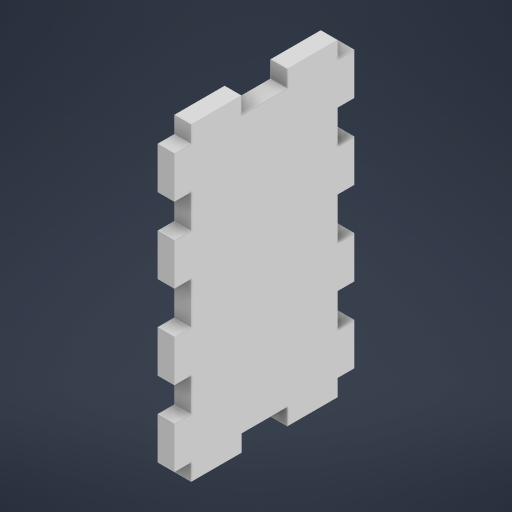
# Autodesk Inventor part: Langbektang houder
Saved by Autodesk Inventor 2023.2 (Build 272271000, 271)
## iProperties
Created: 2020-09-09
Part Number: Langbektang houder
Material: Generic
Document SubType Name: Modeling
Designer: nathan.bollaert
Density: 1 g/cm^3
Appearance: Default
Author: nathan.bollaert
Autodesk Inventor part; units mm, degrees
ref_plane "YZ Plane" through (0, 0, 0) normal (1, 0, 0) x (0, 1, 0)
ref_plane "XZ Plane" through (0, 0, 0) normal (0, 1, 0) x (-1, 0, 0)
ref_plane "XY Plane" through (0, 0, 0) normal (0, 0, 1) x (1, 0, 0)
sketch "Sketch1" plane through (0, 0, 0) normal (1, 0, 0) x (0, 1, 0)
  line L0 (0, 0) -> (74, 0)
  line L1 (74, 0) -> (74, -43)
  line L2 (74, -43) -> (0, -43)
  line L3 (0, -43) -> (0, 0)
  dimension "d228" = 74
  dimension "d229" = 43
  constraints: 8 end point, 2 parallel, 1 horizontal, 1 perpendicular
  measures "d228" distance of L1.end L2.end
  measures "d229" distance of L0.end L1.end
extrude "Extrusion1" add sketch "Sketch1" against normal blind 4
sketch "Sketch15" plane through (0, 0, 0) normal (1, 0, 0) x (0, 0, -1)
  line L0 (0, 74) -> (43, 74) projected
  line L1 (21.5, 74) -> (21.5, 0)
  line L2 (43, 0) -> (0, 0) projected
  line L3 (0, 0) -> (0, 74) projected
  line L4 (0, 37) -> (43, 37)
  line L5 (43, 74) -> (43, 0) projected
  line L6 (0, 70) -> (4, 70)
  line L7 (4, 70) -> (4, 74)
  line L8 (16, 74) -> (16, 70)
  line L9 (16, 70) -> (27, 70)
  line L10 (27, 70) -> (27, 74)
  line L11 (39, 74) -> (39, 70)
  line L12 (39, 70) -> (43, 70)
  line L13 (4, 74) -> (16, 74)
  line L14 (27, 74) -> (39, 74)
  line L15 (0, 0) -> (43, 0)
  line L16 (0, 4) -> (4, 4)
  line L17 (4, 4) -> (4, 0)
  line L18 (16, 0) -> (16, 4)
  line L19 (16, 4) -> (27, 4)
  line L20 (27, 4) -> (27, 0)
  line L21 (39, 0) -> (39, 4)
  line L22 (39, 4) -> (43, 4)
  line L23 (4, 0) -> (16, 0)
  line L24 (27, 0) -> (39, 0)
  line L25 (0, 70) -> (0, 60)
  line L26 (0, 60) -> (4, 60)
  line L27 (4, 60) -> (4, 52)
  line L28 (4, 52) -> (0, 52)
  line L29 (0, 52) -> (0, 42)
  line L30 (0, 42) -> (4, 42)
  line L31 (4, 42) -> (4, 32)
  line L32 (4, 32) -> (0, 32)
  line L33 (0, 32) -> (0, 22)
  line L34 (0, 22) -> (4, 22)
  line L35 (4, 22) -> (4, 14)
  line L36 (4, 14) -> (0, 14)
  line L37 (0, 74) -> (0, 0) projected
  line L38 (43, 0) -> (43, 74)
  line L39 (43, 37) -> (0, 37)
  line L40 (43, 70) -> (43, 60)
  line L41 (43, 60) -> (39, 60)
  line L42 (39, 60) -> (39, 52)
  line L43 (39, 52) -> (43, 52)
  line L44 (43, 52) -> (43, 42)
  line L45 (43, 42) -> (39, 42)
  line L46 (39, 42) -> (39, 32)
  line L47 (39, 32) -> (43, 32)
  line L48 (43, 32) -> (43, 22)
  line L49 (43, 22) -> (39, 22)
  line L50 (39, 22) -> (39, 14)
  line L51 (39, 14) -> (43, 14)
  line L52 (43, 74) -> (43, 0)
  dimension "d232" = 4
  dimension "d233" = 12
  dimension "d234" = 10
  dimension "d246" = 10
  dimension "d248" = 8
  dimension "d250" = 10
  constraints: 92 end point, 24 symmetric about line, 19 point on line, 10 equal length, 7 perpendicular, 3 midpoint, 2 collinear, 2 horizontal, 1 parallel, 1 vertical, 25 other
  measures "d232" length of L7
  measures "d233" distance between parallel lines of L7 L8
  measures "d234" distance of L6.start L25.end
  measures "d246" distance of L29.end L32.end
  measures "d248" distance of L28.end L25.end
  measures "d250" distance of L28.end L29.end
extrude "Extrusion17" cut sketch "Sketch15" against normal blind 4 contours L0 L7 L6 L3 | L0 L1 L9 L8 | L26 L27 L28 L3 | L0 L10 L9 L1 | L30 L31 L4 L3 | L0 L5 L12 L11 | L4 L31 L32 L3 | L19 L20 L2 L1 | L1 L2 L18 L19 | L46 L45 L5 L4 | L4 L5 L47 L46 | L34 L35 L36 L3 | L5 L43 L42 L41 | L21 L22 L5 L2 | L2 L3 L16 L17 | L5 L51 L50 L49
body "Solid5"
